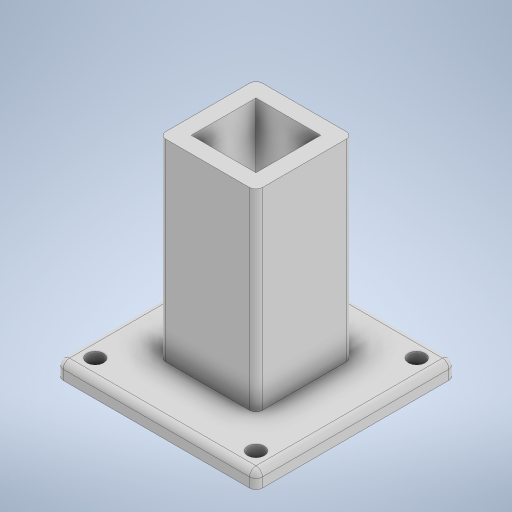
# Autodesk Inventor part: Profile_Holder
Saved by Autodesk Inventor 2024.3 (Build 283343000, 343)
## iProperties
Created: 2025-09-23
Part Number: Profile_Holder
Material: 일반
Document SubType Name: Modeling
Designer: joung
Density: 1 g/cm^3
Appearance: 기본값
Author: joung
Autodesk Inventor part; units mm, degrees
ref_plane "YZ Plane" through (0, 0, 0) normal (1, 0, 0) x (0, 1, 0)
ref_plane "XZ Plane" through (0, 0, 0) normal (0, 1, 0) x (-1, 0, 0)
ref_plane "XY Plane" through (0, 0, 0) normal (0, 0, 1) x (1, 0, 0)
sketch "스케치2" plane through (0, 0, 0) normal (0, 1, 0) x (-1, 0, 0)
  line L0 (25, 25) -> (-25, 25)
  line L1 (-25, 25) -> (-25, -25)
  line L2 (-25, -25) -> (25, -25)
  line L3 (25, -25) -> (25, 25)
  line L4 (25, 25) -> (-25, -25) construction
  line L5 (-25, 25) -> (25, -25) construction
  circle A0 centre (25, -25) radius 2.6
  circle A1 centre (-25, -25) radius 2.6
  circle A2 centre (25, 25) radius 2.6
  circle A3 centre (-25, 25) radius 2.6
  line L6 (31, -31) -> (-31, -31)
  line L7 (-31, -31) -> (-31, 31)
  line L8 (-31, 31) -> (31, 31)
  line L9 (31, 31) -> (31, -31)
  line L10 (10.05, 10.05) -> (-10.05, 10.05)
  line L11 (-10.05, 10.05) -> (-10.05, -10.05)
  line L12 (-10.05, -10.05) -> (10.05, -10.05)
  line L13 (10.05, -10.05) -> (10.05, 10.05)
  line L14 (10.05, 10.05) -> (-10.05, -10.05) construction
  line L15 (-10.05, 10.05) -> (10.05, -10.05) construction
  line L16 (-15.05, -15.05) -> (-15.05, 15.05)
  line L17 (-15.05, 15.05) -> (15.05, 15.05)
  line L18 (15.05, 15.05) -> (15.05, -15.05)
  line L19 (15.05, -15.05) -> (-15.05, -15.05)
  point P0 (0, 0)
  dimension "d16" = 50
  dimension "d17" = 50
  dimension "d18" = 5.2
  dimension "d21" = 50
  dimension "d24" = 50
  dimension "d27" = 6
  dimension "d28" = 20.1
  dimension "d29" = 20.1
  dimension "d30" = 5
  constraints: 40 end point, 8 parallel, 4 centre point, 4 midpoint, 4 perpendicular, 3 horizontal, 1 coincident, 1 vertical, 12 other
  measures "d16" distance of L2.end L1.end
  measures "d17" distance of L0.end L1.end
  measures "d18" diameter of A0
  measures "d21" distance of A0.centre A1.centre
  measures "d24" distance of A0.centre A2.centre
  measures "d27" distance between parallel lines of L2 L6
  measures "d28" distance of L12.end L11.end
  measures "d29" distance of L11.end L10.end
  measures "d30" distance between parallel lines of L11 L16
extrude "돌출2" add sketch "스케치2" along normal blind 5 contours L0 A2 L3 A0 L2 A1 L1 A3 | L6 L7 L8 L9 | L13 L12 L11 L10 | L16 L17 L18 L19
sketch "스케치3" plane through (0, 5, 0) normal (0, 1, 0) x (1, 0, 0)
  line L0 (-10.05, 10.05) -> (10.05, 10.05)
  line L1 (10.05, 10.05) -> (10.05, -10.05)
  line L2 (10.05, -10.05) -> (-10.05, -10.05)
  line L3 (-10.05, -10.05) -> (-10.05, 10.05)
  line L4 (-10.05, 10.05) -> (10.05, -10.05) construction
  line L5 (10.05, 10.05) -> (-10.05, -10.05) construction
  line L6 (15.05, 15.05) -> (-15.05, 15.05)
  line L7 (-15.05, 15.05) -> (-15.05, -15.05)
  line L8 (-15.05, -15.05) -> (15.05, -15.05)
  line L9 (15.05, -15.05) -> (15.05, 15.05)
  point P0 (0, 0)
  dimension "d33" = 20.1
  dimension "d34" = 20.1
  dimension "d35" = 5
  constraints: 20 end point, 4 parallel, 2 midpoint, 2 perpendicular, 1 horizontal, 3 other
  measures "d33" distance of L1.end L2.end
  measures "d34" distance of L0.end L1.end
  measures "d35" distance between parallel lines of L0 L6
extrude "돌출3" add sketch "스케치3" along normal blind 60
fillet "모깎기1" radius 2 12 edges at (-31, 5, 0) (0, 5, -31) (0, 5, 31) (31, 5, 0) (-31, 2.5, -31) (-31, 2.5, 31) (31, 2.5, 31) (31, 2.5, -31) (-15.05, 35, 15.05) (15.05, 35, 15.05) (15.05, 35, -15.05) (-15.05, 35, -15.05)
